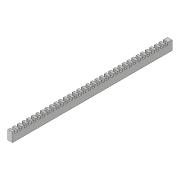
# Autodesk Inventor part: rack
Saved by Autodesk Inventor 2019 (Build 230136000, 136)
## iProperties
Created: 2020-02-12
Part Number: rack
Material: Generic
Document SubType Name: Modeling
Designer: Admin
Density: 1 g/cm^3
Appearance: Default
Author: Admin
Autodesk Inventor part; units mm, degrees
ref_plane "YZ Plane" through (0, 0, 0) normal (1, 0, 0) x (0, 1, 0)
ref_plane "XZ Plane" through (0, 0, 0) normal (0, 1, 0) x (-1, 0, 0)
ref_plane "XY Plane" through (0, 0, 0) normal (0, 0, 1) x (1, 0, 0)
sketch "Sketch1" plane through (0, 0, 0) normal (1, 0, 0) x (0, 1, 0)
  line L0 (0, 0) -> (0, -700)
  line L1 (0, -700) -> (-40, -700)
  line L2 (-40, -700) -> (-40, 0)
  line L3 (-40, 0) -> (0, 0)
  dimension "d0" = 700
  dimension "d1" = 40
  dimension "d2" = 700
  dimension "d3" = 40
  constraints: 8 end point, 2 perpendicular, 1 vertical
  measures "d0" distance of L0.start L0.end
  measures "d1" distance of L0.end L1.end
  measures "d2" distance of L1.end L2.end
  measures "d3" distance of L2.end L0.start
extrude "Extrusion1" add sketch "Sketch1" along normal blind 20
sketch "Sketch2" plane through (20, 0, 0) normal (1, 0, 0) x (0, 0, -1)
  line L0 (700, 0) -> (0, 0) projected
  line L1 (0, 0) -> (10, 0)
  line L2 (10, 0) -> (10, -10)
  line L3 (10, -10) -> (20, -10)
  line L4 (20, -10) -> (20, 0)
  line L5 (20, 0) -> (30, 0)
  line L6 (30, 0) -> (30, -10)
  line L7 (30, -10) -> (40, -10)
  line L8 (40, -10) -> (40, 0)
  line L9 (40, 0) -> (51.6608, 0)
  line L10 (51.6608, 0) -> (51.6608, -10)
  line L11 (51.6608, -10) -> (61.6608, -10)
  line L12 (61.6608, -10) -> (61.6608, 0)
  line L13 (61.6608, 0) -> (71.6608, 0)
  line L14 (71.6608, 0) -> (71.6608, -10)
  line L15 (71.6608, -10) -> (81.6608, -10)
  line L16 (81.6608, -10) -> (81.6608, 0)
  line L17 (81.6608, 0) -> (91.6608, 0)
  line L18 (91.6608, 0) -> (91.6608, -10)
  line L19 (91.6608, -10) -> (101.6608, -10)
  line L20 (101.6608, -10) -> (101.6608, 0)
  line L21 (101.6608, 0) -> (111.6608, 0)
  line L22 (111.6608, 0) -> (111.6608, -10)
  line L23 (111.6608, -10) -> (121.6608, -10)
  line L24 (121.6608, -10) -> (121.6608, 0)
  line L25 (121.6608, 0) -> (131.6608, 0)
  line L26 (131.6608, 0) -> (131.6608, -10)
  line L27 (131.6608, -10) -> (141.6608, -10)
  line L28 (141.6608, -10) -> (141.6608, 0)
  line L29 (141.6608, 0) -> (151.6608, 0)
  line L30 (151.6608, 0) -> (151.6608, -10)
  line L31 (151.6608, -10) -> (161.6608, -10)
  line L32 (161.6608, -10) -> (161.6608, 0)
  line L33 (161.6608, 0) -> (171.6608, 0)
  line L34 (171.6608, 0) -> (171.6608, -10)
  line L35 (171.6608, -10) -> (181.6608, -10)
  line L36 (181.6608, -10) -> (181.6608, 0)
  line L37 (181.6608, 0) -> (191.6608, 0)
  line L38 (191.6608, 0) -> (191.6608, -10)
  line L39 (191.6608, -10) -> (201.6608, -10)
  line L40 (201.6608, -10) -> (201.6608, 0)
  line L41 (0, 0) -> (700, 0)
  dimension "d6" = 10
  dimension "d7" = 10
  dimension "d8" = 10
  dimension "d9" = 10
  dimension "d10" = 10
  dimension "d11" = 10
  dimension "d12" = 10
  dimension "d13" = 10
  dimension "d14" = 10
  dimension "d15" = 10
  dimension "d16" = 10
  dimension "d17" = 10
  dimension "d18" = 10
  dimension "d19" = 10
  dimension "d20" = 10
  dimension "d21" = 10
  dimension "d22" = 10
  dimension "d23" = 10
  dimension "d24" = 10
  dimension "d25" = 10
  dimension "d26" = 10
  dimension "d27" = 10
  dimension "d28" = 10
  dimension "d29" = 10
  dimension "d30" = 10
  dimension "d31" = 10
  dimension "d32" = 10
  dimension "d33" = 10
  dimension "d34" = 10
  dimension "d35" = 10
  dimension "d36" = 10
  dimension "d37" = 10
  dimension "d38" = 10
  dimension "d39" = 10
  dimension "d40" = 10
  dimension "d41" = 10
  dimension "d42" = 10
  dimension "d43" = 10
  dimension "d44" = 10
  dimension "d45" = 700
  constraints: 82 end point, 16 point on line, 3 perpendicular, 1 collinear, 1 vertical, 21 other
  measures "d6" distance of L1.start L1.end
  measures "d7" distance of L1.end L2.end
  measures "d8" distance of L2.end L3.end
  measures "d9" distance of L3.end L4.end
  measures "d10" distance of L4.end L5.end
  measures "d11" distance of L5.end L6.end
  measures "d12" distance of L6.end L7.end
  measures "d13" distance of L7.end L8.end
  measures "d14" distance of L9.end L10.end
  measures "d15" distance of L10.end L11.end
  measures "d16" distance of L11.end L12.end
  measures "d17" distance of L12.end L13.end
  measures "d18" distance of L13.end L14.end
  measures "d19" distance of L14.end L15.end
  measures "d20" distance of L15.end L16.end
  measures "d21" distance of L16.end L17.end
  measures "d22" distance of L17.end L18.end
  measures "d23" distance of L18.end L19.end
  measures "d24" distance of L19.end L20.end
  measures "d25" distance of L20.end L21.end
  measures "d26" distance of L21.end L22.end
  measures "d27" distance of L22.end L23.end
  measures "d28" distance of L23.end L24.end
  measures "d29" distance of L24.end L25.end
  measures "d30" distance of L25.end L26.end
  measures "d31" distance of L26.end L27.end
  measures "d32" distance of L27.end L28.end
  measures "d33" distance of L28.end L29.end
  measures "d34" distance of L29.end L30.end
  measures "d35" distance of L30.end L31.end
  measures "d36" distance of L31.end L32.end
  measures "d37" distance of L32.end L33.end
  measures "d38" distance of L33.end L34.end
  measures "d39" distance of L34.end L35.end
  measures "d40" distance of L35.end L36.end
  measures "d41" distance of L36.end L37.end
  measures "d42" distance of L37.end L38.end
  measures "d43" distance of L38.end L39.end
  measures "d44" distance of L39.end L40.end
  measures "d45" distance of L1.start L41.end
extrude "Extrusion2" cut sketch "Sketch2" against normal blind 40
sketch "Sketch3" plane through (20, 0, 0) normal (1, 0, 0) x (0, 0, -1)
  line L0 (700, 0) -> (201.6608, 0) projected
  line L1 (201.6608, 0) -> (211.6608, 0)
  line L2 (211.6608, 0) -> (211.6608, -10)
  line L3 (211.6608, -10) -> (221.6608, -10)
  line L4 (221.6608, -10) -> (221.6608, 0)
  line L5 (221.6608, 0) -> (231.6608, 0)
  line L6 (231.6608, 0) -> (231.6608, -10)
  line L7 (231.6608, -10) -> (241.6608, -10)
  line L8 (241.6608, -10) -> (241.6608, 0)
  line L9 (241.6608, 0) -> (251.6608, 0)
  line L10 (251.6608, 0) -> (251.6608, -10)
  line L11 (251.6608, -10) -> (261.6608, -10)
  line L12 (261.6608, -10) -> (261.6608, 0)
  line L13 (261.6608, 0) -> (271.6608, 0)
  line L14 (271.6608, 0) -> (271.6608, -10)
  line L15 (271.6608, -10) -> (281.6608, -10)
  line L16 (281.6608, -10) -> (281.6608, 0)
  line L17 (281.6608, 0) -> (291.6608, 0)
  line L18 (291.6608, 0) -> (291.6608, -10)
  line L19 (291.6608, -10) -> (301.6608, -10)
  line L20 (301.6608, -10) -> (301.6608, 0)
  line L21 (301.6608, 0) -> (311.6608, 0)
  line L22 (311.6608, 0) -> (311.6608, -10)
  line L23 (311.6608, -10) -> (321.6608, -10)
  line L24 (321.6608, -10) -> (321.6608, 0)
  line L25 (321.6608, 0) -> (331.6608, 0)
  line L26 (331.6608, 0) -> (331.6608, -10)
  line L27 (331.6608, -10) -> (341.6608, -10)
  line L28 (341.6608, -10) -> (341.6608, 0)
  line L29 (341.6608, 0) -> (351.6608, 0)
  line L30 (351.6608, 0) -> (351.6608, -10)
  line L31 (351.6608, -10) -> (361.6608, -10)
  line L32 (361.6608, -10) -> (361.6608, 0)
  line L33 (361.6608, 0) -> (371.6608, 0)
  line L34 (371.6608, 0) -> (371.6608, -10)
  line L35 (371.6608, -10) -> (381.6608, -10)
  line L36 (381.6608, -10) -> (381.6608, 0)
  line L37 (381.6608, 0) -> (391.6608, 0)
  line L38 (391.6608, 0) -> (391.6608, -10)
  line L39 (391.6608, -10) -> (401.6608, -10)
  line L40 (401.6608, -10) -> (401.6608, 0)
  line L41 (401.6608, 0) -> (411.6608, 0)
  line L42 (411.6608, 0) -> (411.6608, -10)
  line L43 (411.6608, -10) -> (421.6608, -10)
  line L44 (421.6608, -10) -> (421.6608, 0)
  line L45 (421.6608, 0) -> (431.6608, 0)
  line L46 (431.6608, 0) -> (431.6608, -10)
  line L47 (431.6608, -10) -> (441.6608, -10)
  line L48 (441.6608, -10) -> (441.6608, 0)
  line L49 (441.6608, 0) -> (451.6608, 0)
  line L50 (451.6608, 0) -> (451.6608, -10)
  line L51 (451.6608, -10) -> (461.6608, -10)
  line L52 (461.6608, -10) -> (461.6608, 0)
  line L53 (461.6608, 0) -> (471.6608, 0)
  line L54 (471.6608, 0) -> (471.6608, -10)
  line L55 (471.6608, -10) -> (481.6608, -10)
  line L56 (481.6608, -10) -> (481.6608, 0)
  line L57 (481.6608, 0) -> (491.6608, 0)
  line L58 (491.6608, 0) -> (491.6608, -10)
  line L59 (491.6608, -10) -> (501.6608, -10)
  line L60 (501.6608, -10) -> (501.6608, 0)
  line L61 (501.6608, 0) -> (511.6608, 0)
  line L62 (511.6608, 0) -> (511.6608, -10)
  line L63 (511.6608, -10) -> (521.6608, -10)
  line L64 (521.6608, -10) -> (521.6608, 0)
  line L65 (521.6608, 0) -> (531.6608, 0)
  line L66 (531.6608, 0) -> (531.6608, -10)
  line L67 (531.6608, -10) -> (541.6608, -10)
  line L68 (541.6608, -10) -> (541.6608, 0)
  line L69 (541.6608, 0) -> (551.6608, 0)
  line L70 (551.6608, 0) -> (551.6608, -10)
  line L71 (551.6608, -10) -> (561.6608, -10)
  line L72 (561.6608, -10) -> (561.6608, 0)
  line L73 (561.6608, 0) -> (571.6608, 0)
  line L74 (571.6608, 0) -> (571.6608, -10)
  line L75 (571.6608, -10) -> (581.6608, -10)
  line L76 (581.6608, -10) -> (581.6608, 0)
  line L77 (581.6608, 0) -> (591.6608, 0)
  line L78 (591.6608, 0) -> (591.6608, -10)
  line L79 (591.6608, -10) -> (601.6608, -10)
  line L80 (601.6608, -10) -> (601.6608, 0)
  line L81 (601.6608, 0) -> (611.6608, 0)
  line L82 (611.6608, 0) -> (611.6608, -10)
  line L83 (611.6608, -10) -> (621.6608, -10)
  line L84 (621.6608, -10) -> (621.6608, 0)
  line L85 (621.6608, 0) -> (631.6608, 0)
  line L86 (631.6608, 0) -> (631.6608, -10)
  line L87 (631.6608, -10) -> (641.6608, -10)
  line L88 (641.6608, -10) -> (641.6608, 0)
  line L89 (641.6608, 0) -> (651.6608, 0)
  line L90 (651.6608, 0) -> (651.6608, -10)
  line L91 (651.6608, -10) -> (661.6608, -10)
  line L92 (661.6608, -10) -> (661.6608, 0)
  line L93 (661.6608, 0) -> (671.6608, 0)
  line L94 (671.6608, 0) -> (671.6608, -10)
  line L95 (671.6608, -10) -> (681.6608, -10)
  line L96 (681.6608, -10) -> (681.6608, 0)
  line L97 (681.6608, 0) -> (691.6608, 0)
  line L98 (691.6608, 0) -> (691.6608, -10)
  line L99 (691.6608, -10) -> (701.6608, -10)
  line L100 (201.6608, 0) -> (733.4893, 0)
  point P0 (0, 0)
  dimension "d48" = 10
  dimension "d49" = 10
  dimension "d50" = 10
  dimension "d51" = 10
  dimension "d52" = 10
  dimension "d53" = 10
  dimension "d54" = 10
  dimension "d55" = 10
  dimension "d56" = 10
  dimension "d57" = 10
  dimension "d58" = 10
  dimension "d59" = 10
  dimension "d60" = 10
  dimension "d61" = 10
  dimension "d62" = 10
  dimension "d63" = 10
  dimension "d64" = 10
  dimension "d65" = 10
  dimension "d66" = 10
  dimension "d67" = 10
  dimension "d68" = 10
  dimension "d69" = 10
  dimension "d70" = 10
  dimension "d71" = 10
  dimension "d72" = 10
  dimension "d73" = 10
  dimension "d74" = 10
  dimension "d75" = 10
  dimension "d76" = 10
  dimension "d77" = 10
  dimension "d78" = 10
  dimension "d79" = 10
  dimension "d80" = 10
  dimension "d81" = 10
  dimension "d82" = 10
  dimension "d83" = 10
  dimension "d84" = 10
  dimension "d85" = 10
  dimension "d86" = 10
  dimension "d87" = 10
  dimension "d88" = 10
  dimension "d89" = 10
  dimension "d90" = 10
  dimension "d91" = 10
  dimension "d92" = 10
  dimension "d93" = 10
  dimension "d94" = 10
  dimension "d95" = 10
  dimension "d96" = 10
  dimension "d97" = 10
  dimension "d98" = 10
  dimension "d99" = 10
  dimension "d100" = 10
  dimension "d101" = 10
  dimension "d102" = 10
  dimension "d103" = 10
  dimension "d104" = 10
  dimension "d105" = 10
  dimension "d106" = 10
  dimension "d107" = 10
  dimension "d108" = 10
  dimension "d109" = 10
  dimension "d110" = 10
  dimension "d111" = 10
  constraints: 200 end point, 48 point on line, 2 perpendicular, 1 horizontal, 50 other
  measures "d48" distance of L1.start L1.end
  measures "d49" distance of L1.end L2.end
  measures "d50" distance of L2.end L3.end
  measures "d51" distance of L3.end L4.end
  measures "d52" distance of L4.end L5.end
  measures "d53" distance of L5.end L6.end
  measures "d54" distance of L6.end L7.end
  measures "d55" distance of L7.end L8.end
  measures "d56" distance of L8.end L9.end
  measures "d57" distance of L9.end L10.end
  measures "d58" distance of L10.end L11.end
  measures "d59" distance of L11.end L12.end
  measures "d60" distance of L12.end L13.end
  measures "d61" distance of L13.end L14.end
  measures "d62" distance of L14.end L15.end
  measures "d63" distance of L15.end L16.end
  measures "d64" distance of L16.end L17.end
  measures "d65" distance of L17.end L18.end
  measures "d66" distance of L18.end L19.end
  measures "d67" distance of L19.end L20.end
  measures "d68" distance of L20.end L21.end
  measures "d69" distance of L21.end L22.end
  measures "d70" distance of L22.end L23.end
  measures "d71" distance of L23.end L24.end
  measures "d72" distance of L24.end L25.end
  measures "d73" distance of L25.end L26.end
  measures "d74" distance of L26.end L27.end
  measures "d75" distance of L27.end L28.end
  measures "d76" distance of L28.end L29.end
  measures "d77" distance of L29.end L30.end
  measures "d78" distance of L30.end L31.end
  measures "d79" distance of L31.end L32.end
  measures "d80" distance of L32.end L33.end
  measures "d81" distance of L33.end L34.end
  measures "d82" distance of L34.end L35.end
  measures "d83" distance of L35.end L36.end
  measures "d84" distance of L36.end L37.end
  measures "d85" distance of L37.end L38.end
  measures "d86" distance of L38.end L39.end
  measures "d87" distance of L39.end L40.end
  measures "d88" distance of L40.end L41.end
  measures "d89" distance of L41.end L42.end
  measures "d90" distance of L42.end L43.end
  measures "d91" distance of L43.end L44.end
  measures "d92" distance of L44.end L45.end
  measures "d93" distance of L45.end L46.end
  measures "d94" distance of L46.end L47.end
  measures "d95" distance of L47.end L48.end
  measures "d96" distance of L48.end L49.end
  measures "d97" distance of L49.end L50.end
  measures "d98" distance of L50.end L51.end
  measures "d99" distance of L51.end L52.end
  measures "d100" distance of L52.end L53.end
  measures "d101" distance of L53.end L54.end
  measures "d102" distance of L54.end L55.end
  measures "d103" distance of L55.end L56.end
  measures "d104" distance of L56.end L57.end
  measures "d105" distance of L57.end L58.end
  measures "d106" distance of L58.end L59.end
  measures "d107" distance of L59.end L60.end
  measures "d108" distance of L60.end L61.end
  measures "d109" distance of L61.end L62.end
  measures "d110" distance of L62.end L63.end
  measures "d111" distance of L63.end L64.end
extrude "Extrusion3" cut sketch "Sketch3" against normal blind 150
body "Solid1"
